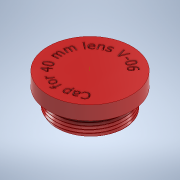
# Autodesk Inventor part: CapForSvBonyPlosse-40mm-V06
Saved by Autodesk Inventor 2021.1 (Build 251245010, 245A)
## iProperties
Created: 2020-10-08
Part Number: CapForSvBonyPlosse-40mm-V06
Material: PC/ABS Plastic
Document SubType Name: Modeling
Designer: robst
Density: 0.357273 g/cm^3
Appearance: Red
Author: robst
Autodesk Inventor part; units mm, degrees
ref_plane "YZ Plane" through (0, 0, 0) normal (1, 0, 0) x (0, 1, 0)
ref_plane "XZ Plane" through (0, 0, 0) normal (0, 1, 0) x (-1, 0, 0)
ref_plane "XY Plane" through (0, 0, 0) normal (0, 0, 1) x (1, 0, 0)
sketch "Sketch7" plane through (0, 0, 0) normal (0, 0, 1) x (1, 0, 0)
  line L0 (0, 0) -> (23.5712, 0)
  line L1 (23.5712, 0) -> (23.5712, 12.7)
  line L2 (23.5712, 12.7) -> (28.575, 12.7)
  line L3 (28.575, 12.7) -> (28.575, 22.225)
  line L4 (28.575, 22.225) -> (0, 22.225)
  line L5 (23.5712, 0) -> (20.3962, 0)
  line L6 (20.3962, 0) -> (20.3962, 19.05)
  line L7 (20.3962, 19.05) -> (12.7, 19.05)
  line L8 (0, 22.225) -> (0, 19.05)
  line L9 (0, -4.445) -> (0, 26.67) projected
  line L10 (0, 19.05) -> (0, 0)
  line L11 (0, 0) -> (12.7, 0)
  line L12 (12.7, 19.05) -> (12.7, 0)
  dimension "d71" = 9.525
  dimension "d72" = 12.7
  dimension "d73" = 23.5712
  dimension "d78" = 3.175
  dimension "d117" = 20.3962
  dimension "d118" = 28.575
  dimension "d122" = 12.7
  constraints: 24 end point, 6 perpendicular, 2 point on line, 2 vertical, 1 collinear, 1 horizontal
  measures "d71" distance between parallel lines of L4 L2
  measures "d72" distance from line of L2 L0.start
  measures "d73" distance of L0.start L0.end
  measures "d78" distance between parallel lines of L1 L6
  measures "d117" distance between parallel lines of L6 L9
  measures "d118" distance from line of L3 L0.start
  measures "d122" distance between parallel lines of L12 L9
revolve "Revolution3" add sketch "Sketch7" angle 360 about axis through (0, -10, 0) along (0, 1, 0) contours L9 L8 L4 L3 L2 L1 L0 L6 L7 L12
sketch "Sketch10" plane through (0, 0, 0) normal (0, 0, 1) x (1, 0, 0)
  line L0 (23.5712, 12.7) -> (23.5712, 0) projected
  line L1 (23.5712, -2.1167) -> (23.5712, -4.0025)
  line L2 (23.5712, -4.0025) -> (22.3266, -3.284)
  line L3 (22.3266, -2.8352) -> (23.5712, -2.1167)
  line L4 (-23.5712, 0) -> (23.5712, 0) projected
  arc A0 (22.3266, -2.8352) -> (22.3266, -3.284) centre (22.4561, -3.0596) ccw
  line L5 (0, -7.3431) -> (0, 16.0405) projected
  point P0 (0, 0)
  dimension "d100" = 60
  dimension "d101" = 2.1167
  dimension "d102" = 0.2591
  dimension "d103" = 22.1971
  constraints: 6 end point, 2 point on circle, 2 tangent, 1 centre point, 1 collinear, 1 equal length, 1 vertical
  measures "d100" angle of L3 L2
  measures "d101" distance from line of L1.start L4
  measures "d102" radius of A0
  measures "d103" distance edge to line of A0 L5
coil "Coil6" sketch "Sketch10" operation cut axis through (0, -10, 0) along (0, 1, 0) pitch 2.1167 turns 8 hand right
sketch "Sketch11" plane through (0, 22.225, 0) normal (0, 1, 0) x (1, 0, 0)
  circle A0 centre (0, 0) radius 20.955 construction
  circle A1 centre (0, 0) radius 28.575 projected
  spline S0 degree 2 poles (11.1336, -14.1453) (11.5615, -13.7907) (12.5248, -13.4798) (13.028, -13.55) knots 0 0 0 1 2 2 2
  spline S1 degree 2 poles (13.028, -13.55) (13.5283, -13.6166) (14.5263, -14.2332) (14.9873, -14.7895) knots 0 0 0 1 2 2 2
  spline S2 degree 2 poles (14.9873, -14.7895) (15.4453, -15.3423) (15.8431, -16.396) (15.8268, -16.9207) knots 0 0 0 1 2 2 2
  spline S3 degree 2 poles (15.8268, -16.9207) (15.8082, -17.4354) (15.3448, -18.3425) (14.8991, -18.7118) knots 0 0 0 1 2 2 2
  spline S4 degree 2 poles (14.8991, -18.7118) (14.678, -18.895) (14.2361, -19.1529) (14.0306, -19.2389) knots 0 0 0 1 2 2 2
  spline S5 degree 2 poles (14.0306, -19.2389) (13.8496, -19.3107) (13.4443, -19.424) (13.233, -19.4667) knots 0 0 0 1 2 2 2
  line L0 (13.233, -19.4667) -> (12.648, -18.7606)
  line L1 (12.648, -18.7606) -> (12.6943, -18.7222)
  spline S6 degree 2 poles (12.6943, -18.7222) (12.8319, -18.7285) (13.2399, -18.7273) (13.4944, -18.6788) knots 0 0 0 1 2 2 2
  spline S7 degree 2 poles (13.4944, -18.6788) (13.7388, -18.6326) (14.2322, -18.4223) (14.489, -18.2096) knots 0 0 0 1 2 2 2
  spline S8 degree 2 poles (14.489, -18.2096) (14.7707, -17.9762) (15.0815, -17.3277) (15.0873, -16.95) knots 0 0 0 1 2 2 2
  spline S9 degree 2 poles (15.0873, -16.95) (15.0866, -16.5717) (14.7291, -15.7192) (14.3774, -15.2948) knots 0 0 0 1 2 2 2
  spline S10 degree 2 poles (14.3774, -15.2948) (14.0022, -14.8419) (13.2439, -14.3695) (12.8688, -14.3014) knots 0 0 0 1 2 2 2
  spline S11 degree 2 poles (12.8688, -14.3014) (12.5031, -14.2375) (11.8242, -14.4272) (11.546, -14.6576) knots 0 0 0 1 2 2 2
  spline S12 degree 2 poles (11.546, -14.6576) (11.2928, -14.8674) (10.9647, -15.3498) (10.8739, -15.5814) knots 0 0 0 1 2 2 2
  spline S13 degree 2 poles (10.8739, -15.5814) (10.7903, -15.807) (10.7109, -16.1976) (10.6993, -16.3215) knots 0 0 0 1 2 2 2
  line L2 (10.6993, -16.3215) -> (10.6565, -16.3569)
  line L3 (10.6565, -16.3569) -> (10.0773, -15.658)
  spline S14 degree 2 poles (10.0773, -15.658) (10.1674, -15.4691) (10.3208, -15.1315) (10.4554, -14.9237) knots 0 0 0 1 2 2 2
  spline S15 degree 2 poles (10.4554, -14.9237) (10.5948, -14.7) (10.8697, -14.364) (11.1336, -14.1453) knots 0 0 0 1 2 2 2
  spline S16 degree 2 poles (7.2823, -17.0834) (7.3335, -16.9868) (7.5001, -16.6496) (7.5951, -16.5267) knots 0 0 0 1 2 2 2
  spline S17 degree 2 poles (7.5951, -16.5267) (7.722, -16.3526) (7.9971, -16.1019) (8.2892, -15.9612) knots 0 0 0 1 2 2 2
  spline S18 degree 2 poles (8.2892, -15.9612) (8.5271, -15.8467) (9.0432, -15.8192) (9.2843, -15.9036) knots 0 0 0 1 2 2 2
  spline S19 degree 2 poles (9.2843, -15.9036) (9.5151, -15.9878) (9.9279, -16.3647) (10.0524, -16.6234) knots 0 0 0 1 2 2 2
  spline S20 degree 2 poles (10.0524, -16.6234) (10.2453, -17.024) (10.1806, -17.7543) (9.8917, -18.0938) knots 0 0 0 1 2 2 2
  spline S21 degree 2 poles (9.8917, -18.0938) (9.6386, -18.4008) (8.8082, -18.9394) (8.309, -19.2157) knots 0 0 0 1 2 2 2
  line L4 (8.309, -19.2157) -> (8.3693, -19.3409)
  spline S22 degree 2 poles (8.3693, -19.3409) (8.4778, -19.5662) (8.7501, -19.7795) (8.9135, -19.7985) knots 0 0 0 1 2 2 2
  spline S23 degree 2 poles (8.9135, -19.7985) (9.0768, -19.8175) (9.4598, -19.6948) (9.6517, -19.6024) knots 0 0 0 1 2 2 2
  spline S24 degree 2 poles (9.6517, -19.6024) (9.8771, -19.4939) (10.422, -19.067) (10.6643, -18.791) knots 0 0 0 1 2 2 2
  line L5 (10.6643, -18.791) -> (10.7019, -18.7729)
  line L6 (10.7019, -18.7729) -> (11.0213, -19.4364)
  spline S25 degree 2 poles (11.0213, -19.4364) (10.866, -19.5728) (10.2545, -20.0215) (9.9248, -20.1802) knots 0 0 0 1 2 2 2
  spline S26 degree 2 poles (9.9248, -20.1802) (9.5242, -20.3731) (8.9173, -20.5111) (8.622, -20.4528) knots 0 0 0 1 2 2 2
  spline S27 degree 2 poles (8.622, -20.4528) (8.3328, -20.3968) (7.8811, -19.9923) (7.7063, -19.6293) knots 0 0 0 1 2 2 2
  line L7 (7.7063, -19.6293) -> (6.4345, -16.9879)
  line L8 (6.4345, -16.9879) -> (7.0854, -16.6745)
  line L9 (7.0854, -16.6745) -> (7.2823, -17.0834)
  line L10 (7.5435, -17.6259) -> (8.0599, -18.6983)
  spline S28 degree 2 poles (8.0599, -18.6983) (8.2835, -18.5649) (8.9546, -18.1544) (9.1436, -17.9812) knots 0 0 0 1 2 2 2
  spline S29 degree 2 poles (9.1436, -17.9812) (9.3641, -17.7773) (9.5434, -17.2849) (9.4027, -16.9928) knots 0 0 0 1 2 2 2
  spline S30 degree 2 poles (9.4027, -16.9928) (9.242, -16.659) (8.7037, -16.5018) (8.3448, -16.6746) knots 0 0 0 1 2 2 2
  spline S31 degree 2 poles (8.3448, -16.6746) (8.0402, -16.8213) (7.6661, -17.3253) (7.5435, -17.6259) knots 0 0 0 1 2 2 2
  spline S32 degree 2 poles (2.4585, -20.302) (2.2284, -19.2524) (2.9565, -17.7937) (3.7211, -17.6262) knots 0 0 0 1 2 2 2
  spline S33 degree 2 poles (3.7211, -17.6262) (4.0332, -17.5578) (4.5445, -17.5974) (4.826, -17.6922) knots 0 0 0 1 2 2 2
  line L11 (4.826, -17.6922) -> (4.4413, -15.9369)
  line L12 (4.4413, -15.9369) -> (5.147, -15.7822)
  line L13 (5.147, -15.7822) -> (6.4033, -21.514)
  line L14 (6.4033, -21.514) -> (5.6976, -21.6687)
  line L15 (5.6976, -21.6687) -> (5.6014, -21.2299)
  spline S34 degree 2 poles (5.6014, -21.2299) (5.3916, -21.5271) (4.8186, -21.9846) (4.4431, -22.0669) knots 0 0 0 1 2 2 2
  spline S35 degree 2 poles (4.4431, -22.0669) (3.7238, -22.2246) (2.6687, -21.261) (2.4585, -20.302) knots 0 0 0 1 2 2 2
  spline S36 degree 2 poles (3.169, -20.0609) (3.3266, -20.7802) (3.9571, -21.4717) (4.4683, -21.3597) knots 0 0 0 1 2 2 2
  spline S37 degree 2 poles (4.4683, -21.3597) (4.7668, -21.2942) (5.2693, -20.9044) (5.4725, -20.6418) knots 0 0 0 1 2 2 2
  line L16 (5.4725, -20.6418) -> (4.9509, -18.2622)
  spline S38 degree 2 poles (4.9509, -18.2622) (4.6462, -18.1915) (4.2308, -18.1782) (3.9775, -18.2337) knots 0 0 0 1 2 2 2
  spline S39 degree 2 poles (3.9775, -18.2337) (3.4301, -18.3537) (3.0004, -19.2918) (3.169, -20.0609) knots 0 0 0 1 2 2 2
  line L17 (-4.0637, -23.0619) -> (-4.0269, -23.066)
  spline S40 degree 2 poles (-4.0269, -23.066) (-3.9344, -23.1138) (-3.5827, -23.2188) (-3.4401, -23.235) knots 0 0 0 1 2 2 2
  spline S41 degree 2 poles (-3.4401, -23.235) (-2.9891, -23.286) (-2.5567, -22.9248) (-2.4963, -22.3909) knots 0 0 0 1 2 2 2
  line L18 (-2.4963, -22.3909) -> (-2.4802, -22.2483)
  line L19 (-2.4802, -22.2483) -> (-3.6675, -22.1139)
  line L20 (-3.6675, -22.1139) -> (-3.6003, -21.5203)
  line L21 (-3.6003, -21.5203) -> (-2.436, -21.652)
  line L22 (-2.436, -21.652) -> (-2.021, -17.9843)
  line L23 (-2.021, -17.9843) -> (-1.3031, -18.0655)
  line L24 (-1.3031, -18.0655) -> (-1.7181, -21.7333)
  line L25 (-1.7181, -21.7333) -> (-1.2349, -21.7879)
  line L26 (-1.2349, -21.7879) -> (-1.3021, -22.3816)
  line L27 (-1.3021, -22.3816) -> (-1.7853, -22.3269)
  line L28 (-1.7853, -22.3269) -> (-1.8014, -22.4696)
  spline S42 degree 2 poles (-1.8014, -22.4696) (-1.8878, -23.2335) (-2.7194, -23.9504) (-3.4096, -23.8723) knots 0 0 0 1 2 2 2
  spline S43 degree 2 poles (-3.4096, -23.8723) (-3.6075, -23.8499) (-3.9848, -23.7653) (-4.1381, -23.7199) knots 0 0 0 1 2 2 2
  line L29 (-4.1381, -23.7199) -> (-4.0637, -23.0619)
  spline S44 degree 2 poles (-7.8779, -18.744) (-7.5539, -17.7098) (-6.2065, -16.8943) (-5.3757, -17.1545) knots 0 0 0 1 2 2 2
  spline S45 degree 2 poles (-5.3757, -17.1545) (-4.5227, -17.4217) (-3.91, -18.89) (-4.2229, -19.8888) knots 0 0 0 1 2 2 2
  spline S46 degree 2 poles (-4.2229, -19.8888) (-4.5441, -20.9141) (-5.9075, -21.7343) (-6.7295, -21.4769) knots 0 0 0 1 2 2 2
  spline S47 degree 2 poles (-6.7295, -21.4769) (-7.5604, -21.2166) (-8.2004, -19.7737) (-7.8779, -18.744) knots 0 0 0 1 2 2 2
  spline S48 degree 2 poles (-7.1663, -18.9668) (-7.4155, -19.7624) (-7.0788, -20.7171) (-6.544, -20.8846) knots 0 0 0 1 2 2 2
  spline S49 degree 2 poles (-6.544, -20.8846) (-6.0093, -21.0521) (-5.1836, -20.4614) (-4.9344, -19.6659) knots 0 0 0 1 2 2 2
  spline S50 degree 2 poles (-4.9344, -19.6659) (-4.6922, -18.8925) (-5.0264, -17.9143) (-5.5612, -17.7468) knots 0 0 0 1 2 2 2
  spline S51 degree 2 poles (-5.5612, -17.7468) (-6.0915, -17.5806) (-6.9199, -18.1802) (-7.1663, -18.9668) knots 0 0 0 1 2 2 2
  line L30 (-11.5545, -18.3168) -> (-11.5219, -18.3345)
  spline S52 degree 2 poles (-11.5219, -18.3345) (-11.4598, -18.3948) (-11.3057, -18.4893) (-11.1959, -18.5492) knots 0 0 0 1 2 2 2
  spline S53 degree 2 poles (-11.1959, -18.5492) (-10.9397, -18.6888) (-10.3135, -18.7399) (-9.9661, -18.6445) knots 0 0 0 1 2 2 2
  line L31 (-9.9661, -18.6445) -> (-8.51, -15.9727)
  line L32 (-8.51, -15.9727) -> (-7.8756, -16.3185)
  line L33 (-7.8756, -16.3185) -> (-9.9279, -20.0841)
  line L34 (-9.9279, -20.0841) -> (-10.5623, -19.7384)
  line L35 (-10.5623, -19.7384) -> (-10.2564, -19.1772)
  spline S54 degree 2 poles (-10.2564, -19.1772) (-10.7705, -19.2979) (-11.4244, -19.2685) (-11.6684, -19.1355) knots 0 0 0 1 2 2 2
  spline S55 degree 2 poles (-11.6684, -19.1355) (-11.766, -19.0823) (-11.8592, -19.021) (-11.9135, -18.9756) knots 0 0 0 1 2 2 2
  line L36 (-11.9135, -18.9756) -> (-11.5545, -18.3168)
  line L37 (-16.1257, -12.0919) -> (-15.6665, -12.5945)
  line L38 (-15.6665, -12.5945) -> (-14.2168, -11.27)
  line L39 (-14.2168, -11.27) -> (-13.7201, -11.8136)
  line L40 (-13.7201, -11.8136) -> (-15.1698, -13.1381)
  line L41 (-15.1698, -13.1381) -> (-13.4674, -15.0016)
  line L42 (-13.4674, -15.0016) -> (-14.0623, -15.5451)
  line L43 (-14.0623, -15.5451) -> (-17.9612, -15.6445)
  line L44 (-17.9612, -15.6445) -> (-18.436, -15.1248)
  line L45 (-18.436, -15.1248) -> (-16.1213, -13.0099)
  line L46 (-16.1213, -13.0099) -> (-16.5805, -12.5073)
  line L47 (-16.5805, -12.5073) -> (-16.1257, -12.0919)
  line L48 (-15.6246, -13.5536) -> (-17.2726, -15.0593)
  line L49 (-17.2726, -15.0593) -> (-14.3282, -14.9725)
  line L50 (-14.3282, -14.9725) -> (-15.6246, -13.5536)
  spline S56 degree 2 poles (-19.2293, -8.5261) (-17.8832, -7.7829) (-16.1903, -7.8693) (-15.7404, -8.6843) knots 0 0 0 1 2 2 2
  spline S57 degree 2 poles (-15.7404, -8.6843) (-15.2837, -9.5114) (-16.1415, -10.9953) (-17.4592, -11.7228) knots 0 0 0 1 2 2 2
  spline S58 degree 2 poles (-17.4592, -11.7228) (-18.8134, -12.4704) (-20.4982, -12.3795) (-20.9504, -11.5605) knots 0 0 0 1 2 2 2
  spline S59 degree 2 poles (-20.9504, -11.5605) (-21.4047, -10.7374) (-20.5348, -9.2468) (-19.2293, -8.5261) knots 0 0 0 1 2 2 2
  spline S60 degree 2 poles (-17.2303, -8.544) (-17.5313, -8.5832) (-18.3383, -8.9229) (-18.8532, -9.2072) knots 0 0 0 1 2 2 2
  spline S61 degree 2 poles (-18.8532, -9.2072) (-19.3682, -9.4915) (-20.0816, -9.9911) (-20.2811, -10.2335) knots 0 0 0 1 2 2 2
  spline S62 degree 2 poles (-20.2811, -10.2335) (-20.4805, -10.4759) (-20.5493, -10.9741) (-20.3949, -11.2539) knots 0 0 0 1 2 2 2
  spline S63 degree 2 poles (-20.3949, -11.2539) (-20.2405, -11.5336) (-19.7777, -11.749) (-19.456, -11.7089) knots 0 0 0 1 2 2 2
  spline S64 degree 2 poles (-19.456, -11.7089) (-19.1446, -11.6693) (-18.3258, -11.3125) (-17.8352, -11.0416) knots 0 0 0 1 2 2 2
  spline S65 degree 2 poles (-17.8352, -11.0416) (-17.3082, -10.7507) (-16.6385, -10.2963) (-16.421, -10.0387) knots 0 0 0 1 2 2 2
  spline S66 degree 2 poles (-16.421, -10.0387) (-16.2152, -9.7981) (-16.1347, -9.2829) (-16.2958, -8.9909) knots 0 0 0 1 2 2 2
  spline S67 degree 2 poles (-16.2958, -8.9909) (-16.448, -8.7152) (-16.9108, -8.4999) (-17.2303, -8.544) knots 0 0 0 1 2 2 2
  line L51 (-18.1997, 0.8026) -> (-20.6758, 0.6272)
  spline S68 degree 2 poles (-20.6758, 0.6272) (-20.9715, 0.6062) (-21.4718, 0.5244) (-21.6051, 0.4407) knots 0 0 0 1 2 2 2
  spline S69 degree 2 poles (-21.6051, 0.4407) (-21.7524, 0.3559) (-21.8802, 0.0637) (-21.8629, -0.1812) knots 0 0 0 1 2 2 2
  spline S70 degree 2 poles (-21.8629, -0.1812) (-21.8472, -0.4029) (-21.5386, -0.8918) (-21.2609, -1.1414) knots 0 0 0 1 2 2 2
  spline S71 degree 2 poles (-21.2609, -1.1414) (-21.1966, -1.1322) (-21.0171, -1.1102) (-20.897, -1.1017) knots 0 0 0 1 2 2 2
  line L52 (-20.897, -1.1017) -> (-18.0789, -0.9021)
  line L53 (-18.0789, -0.9021) -> (-18.0279, -1.6228)
  line L54 (-18.0279, -1.6228) -> (-20.5041, -1.7982)
  spline S72 degree 2 poles (-20.5041, -1.7982) (-20.7997, -1.8191) (-21.3, -1.901) (-21.4334, -1.9847) knots 0 0 0 1 2 2 2
  spline S73 degree 2 poles (-21.4334, -1.9847) (-21.5806, -2.0694) (-21.7084, -2.3617) (-21.6911, -2.6065) knots 0 0 0 1 2 2 2
  spline S74 degree 2 poles (-21.6911, -2.6065) (-21.6747, -2.8375) (-21.3474, -3.3297) (-21.104, -3.5539) knots 0 0 0 1 2 2 2
  line L55 (-21.104, -3.5539) -> (-17.9072, -3.3274)
  line L56 (-17.9072, -3.3274) -> (-17.8561, -4.0481)
  line L57 (-17.8561, -4.0481) -> (-22.134, -4.3511)
  line L58 (-22.134, -4.3511) -> (-22.185, -3.6304)
  line L59 (-22.185, -3.6304) -> (-21.7138, -3.5971)
  spline S75 degree 2 poles (-21.7138, -3.5971) (-22.0156, -3.3352) (-22.3643, -2.8028) (-22.3879, -2.4702) knots 0 0 0 1 2 2 2
  spline S76 degree 2 poles (-22.3879, -2.4702) (-22.4147, -2.0913) (-22.1098, -1.4801) (-21.7279, -1.2998) knots 0 0 0 1 2 2 2
  spline S77 degree 2 poles (-21.7279, -1.2998) (-22.1161, -0.9977) (-22.5342, -0.4052) (-22.5597, -0.0448) knots 0 0 0 1 2 2 2
  spline S78 degree 2 poles (-22.5597, -0.0448) (-22.5793, 0.2324) (-22.4405, 0.6972) (-22.2582, 0.8773) knots 0 0 0 1 2 2 2
  spline S79 degree 2 poles (-22.2582, 0.8773) (-22.0763, 1.0619) (-21.5076, 1.2926) (-21.0687, 1.3236) knots 0 0 0 1 2 2 2
  line L60 (-21.0687, 1.3236) -> (-18.2507, 1.5232)
  line L61 (-18.2507, 1.5232) -> (-18.1997, 0.8026)
  line L62 (-16.7452, 7.1742) -> (-19.124, 7.884)
  spline S80 degree 2 poles (-19.124, 7.884) (-19.408, 7.9688) (-19.905, 8.0688) (-20.0593, 8.0375) knots 0 0 0 1 2 2 2
  spline S81 degree 2 poles (-20.0593, 8.0375) (-20.2269, 8.0102) (-20.4497, 7.7819) (-20.5199, 7.5466) knots 0 0 0 1 2 2 2
  spline S82 degree 2 poles (-20.5199, 7.5466) (-20.5835, 7.3336) (-20.4673, 6.7673) (-20.2956, 6.4358) knots 0 0 0 1 2 2 2
  spline S83 degree 2 poles (-20.2956, 6.4358) (-20.2321, 6.4217) (-20.0564, 6.3789) (-19.941, 6.3445) knots 0 0 0 1 2 2 2
  line L63 (-19.941, 6.3445) -> (-17.2339, 5.5366)
  line L64 (-17.2339, 5.5366) -> (-17.4405, 4.8443)
  line L65 (-17.4405, 4.8443) -> (-19.8192, 5.5541)
  spline S84 degree 2 poles (-19.8192, 5.5541) (-20.1032, 5.6389) (-20.6002, 5.7389) (-20.7545, 5.7076) knots 0 0 0 1 2 2 2
  spline S85 degree 2 poles (-20.7545, 5.7076) (-20.9222, 5.6803) (-21.145, 5.452) (-21.2152, 5.2167) knots 0 0 0 1 2 2 2
  spline S86 degree 2 poles (-21.2152, 5.2167) (-21.2814, 4.9948) (-21.1488, 4.4188) (-21.0002, 4.1231) knots 0 0 0 1 2 2 2
  line L66 (-21.0002, 4.1231) -> (-17.9292, 3.2067)
  line L67 (-17.9292, 3.2067) -> (-18.1358, 2.5144)
  line L68 (-18.1358, 2.5144) -> (-22.2453, 3.7407)
  line L69 (-22.2453, 3.7407) -> (-22.0387, 4.433)
  line L70 (-22.0387, 4.433) -> (-21.586, 4.298)
  spline S87 degree 2 poles (-21.586, 4.298) (-21.7759, 4.6495) (-21.9144, 5.2707) (-21.819, 5.5903) knots 0 0 0 1 2 2 2
  spline S88 degree 2 poles (-21.819, 5.5903) (-21.7104, 5.9542) (-21.2094, 6.4185) (-20.7885, 6.4523) knots 0 0 0 1 2 2 2
  spline S89 degree 2 poles (-20.7885, 6.4523) (-21.045, 6.8721) (-21.227, 7.574) (-21.1237, 7.9202) knots 0 0 0 1 2 2 2
  spline S90 degree 2 poles (-21.1237, 7.9202) (-21.0443, 8.1864) (-20.7503, 8.5723) (-20.5162, 8.6765) knots 0 0 0 1 2 2 2
  spline S91 degree 2 poles (-20.5162, 8.6765) (-20.2808, 8.7851) (-19.6674, 8.8002) (-19.2458, 8.6744) knots 0 0 0 1 2 2 2
  line L71 (-19.2458, 8.6744) -> (-16.5387, 7.8665)
  line L72 (-16.5387, 7.8665) -> (-16.7452, 7.1742)
  line L73 (-14.1279, 11.3161) -> (-14.5682, 10.7433)
  line L74 (-14.5682, 10.7433) -> (-19.3011, 14.3816)
  line L75 (-19.3011, 14.3816) -> (-18.8608, 14.9544)
  line L76 (-18.8608, 14.9544) -> (-14.1279, 11.3161)
  spline S92 degree 2 poles (-12.0649, 13.3622) (-12.8157, 12.6598) (-14.4288, 12.73) (-15.1564, 13.5079) knots 0 0 0 1 2 2 2
  spline S93 degree 2 poles (-15.1564, 13.5079) (-15.8715, 14.2723) (-15.9178, 15.9285) (-15.2718, 16.5328) knots 0 0 0 1 2 2 2
  spline S94 degree 2 poles (-15.2718, 16.5328) (-14.9809, 16.8049) (-14.3729, 17.0566) (-14.0395, 17.0324) knots 0 0 0 1 2 2 2
  spline S95 degree 2 poles (-14.0395, 17.0324) (-13.7027, 17.0113) (-13.0394, 16.6615) (-12.6882, 16.2861) knots 0 0 0 1 2 2 2
  line L77 (-12.6882, 16.2861) -> (-12.4193, 15.9986)
  line L78 (-12.4193, 15.9986) -> (-14.5873, 13.9706)
  spline S96 degree 2 poles (-14.5873, 13.9706) (-14.0779, 13.4261) (-12.989, 13.3602) (-12.5019, 13.8158) knots 0 0 0 1 2 2 2
  spline S97 degree 2 poles (-12.5019, 13.8158) (-12.3294, 13.9772) (-12.0674, 14.3682) (-11.989, 14.5556) knots 0 0 0 1 2 2 2
  spline S98 degree 2 poles (-11.989, 14.5556) (-11.9103, 14.7561) (-11.8248, 15.058) (-11.8112, 15.1722) knots 0 0 0 1 2 2 2
  line L79 (-11.8112, 15.1722) -> (-11.7807, 15.2007)
  line L80 (-11.7807, 15.2007) -> (-11.2429, 14.6257)
  spline S99 degree 2 poles (-11.2429, 14.6257) (-11.2994, 14.5031) (-11.4755, 14.1355) (-11.5553, 14.0038) knots 0 0 0 1 2 2 2
  spline S100 degree 2 poles (-11.5553, 14.0038) (-11.6663, 13.8174) (-11.8755, 13.5393) (-12.0649, 13.3622) knots 0 0 0 1 2 2 2
  spline S101 degree 2 poles (-13.3099, 15.9202) (-13.5159, 16.1269) (-13.8949, 16.3558) (-14.0776, 16.3816) knots 0 0 0 1 2 2 2
  spline S102 degree 2 poles (-14.0776, 16.3816) (-14.2796, 16.4145) (-14.6842, 16.2707) (-14.8973, 16.0714) knots 0 0 0 1 2 2 2
  spline S103 degree 2 poles (-14.8973, 16.0714) (-15.107, 15.8753) (-15.2841, 15.4749) (-15.292, 15.2392) knots 0 0 0 1 2 2 2
  spline S104 degree 2 poles (-15.292, 15.2392) (-15.2933, 15.0034) (-15.1335, 14.5884) (-14.9638, 14.3731) knots 0 0 0 1 2 2 2
  line L81 (-14.9638, 14.3731) -> (-13.3099, 15.9202)
  line L82 (-7.4811, 16.5663) -> (-8.1089, 16.2086)
  line L83 (-8.1089, 16.2086) -> (-9.3193, 18.3334)
  spline S105 degree 2 poles (-9.3193, 18.3334) (-9.466, 18.5909) (-9.7665, 19.0061) (-9.9146, 19.0976) knots 0 0 0 1 2 2 2
  spline S106 degree 2 poles (-9.9146, 19.0976) (-10.0712, 19.1949) (-10.4228, 19.1758) (-10.6562, 19.0429) knots 0 0 0 1 2 2 2
  spline S107 degree 2 poles (-10.6562, 19.0429) (-10.8896, 18.9099) (-11.2425, 18.3784) (-11.3653, 18.042) knots 0 0 0 1 2 2 2
  line L84 (-11.3653, 18.042) -> (-9.7789, 15.2573)
  line L85 (-9.7789, 15.2573) -> (-10.4067, 14.8997)
  line L86 (-10.4067, 14.8997) -> (-12.5295, 18.626)
  line L87 (-12.5295, 18.626) -> (-11.9017, 18.9836)
  line L88 (-11.9017, 18.9836) -> (-11.6656, 18.5691)
  spline S108 degree 2 poles (-11.6656, 18.5691) (-11.5283, 18.9831) (-11.1364, 19.5582) (-10.8305, 19.7324) knots 0 0 0 1 2 2 2
  spline S109 degree 2 poles (-10.8305, 19.7324) (-10.2832, 20.0442) (-9.2509, 19.6729) (-8.8589, 18.9848) knots 0 0 0 1 2 2 2
  line L89 (-8.8589, 18.9848) -> (-7.4811, 16.5663)
  spline S110 degree 2 poles (-5.4004, 17.1663) (-5.8118, 17.0387) (-6.5925, 17.039) (-6.8654, 17.0901) knots 0 0 0 1 2 2 2
  line L90 (-6.8654, 17.0901) -> (-7.1055, 17.8642)
  line L91 (-7.1055, 17.8642) -> (-7.0701, 17.8752)
  spline S111 degree 2 poles (-7.0701, 17.8752) (-6.9597, 17.8318) (-6.6687, 17.7378) (-6.4408, 17.7067) knots 0 0 0 1 2 2 2
  spline S112 degree 2 poles (-6.4408, 17.7067) (-6.2423, 17.6762) (-5.7792, 17.684) (-5.5536, 17.754) knots 0 0 0 1 2 2 2
  spline S113 degree 2 poles (-5.5536, 17.754) (-5.3899, 17.8048) (-5.0373, 17.9966) (-4.968, 18.086) knots 0 0 0 1 2 2 2
  spline S114 degree 2 poles (-4.968, 18.086) (-4.8658, 18.2098) (-4.8098, 18.4357) (-4.8702, 18.6303) knots 0 0 0 1 2 2 2
  spline S115 degree 2 poles (-4.8702, 18.6303) (-4.9457, 18.8736) (-5.2893, 19.0434) (-5.6559, 19.0218) knots 0 0 0 1 2 2 2
  spline S116 degree 2 poles (-5.6559, 19.0218) (-5.7982, 19.0116) (-6.2503, 18.9683) (-6.4468, 18.9607) knots 0 0 0 1 2 2 2
  spline S117 degree 2 poles (-6.4468, 18.9607) (-6.9582, 18.9524) (-7.5585, 19.3869) (-7.6833, 19.7894) knots 0 0 0 1 2 2 2
  spline S118 degree 2 poles (-7.6833, 19.7894) (-7.8562, 20.3467) (-7.2357, 21.3005) (-6.5456, 21.5146) knots 0 0 0 1 2 2 2
  spline S119 degree 2 poles (-6.5456, 21.5146) (-6.205, 21.6203) (-5.4628, 21.6662) (-5.1886, 21.6107) knots 0 0 0 1 2 2 2
  line L92 (-5.1886, 21.6107) -> (-4.9595, 20.872)
  line L93 (-4.9595, 20.872) -> (-4.9948, 20.861)
  spline S120 degree 2 poles (-4.9948, 20.861) (-5.3261, 20.991) (-6.0474, 21.0339) (-6.3791, 20.931) knots 0 0 0 1 2 2 2
  spline S121 degree 2 poles (-6.3791, 20.931) (-6.7197, 20.8254) (-7.0994, 20.3924) (-7.0102, 20.1049) knots 0 0 0 1 2 2 2
  spline S122 degree 2 poles (-7.0102, 20.1049) (-6.9293, 19.8439) (-6.5724, 19.6782) (-6.238, 19.6947) knots 0 0 0 1 2 2 2
  spline S123 degree 2 poles (-6.238, 19.6947) (-6.0753, 19.7015) (-5.6702, 19.7399) (-5.4472, 19.7557) knots 0 0 0 1 2 2 2
  spline S124 degree 2 poles (-5.4472, 19.7557) (-4.9603, 19.7807) (-4.337, 19.397) (-4.1957, 18.9414) knots 0 0 0 1 2 2 2
  spline S125 degree 2 poles (-4.1957, 18.9414) (-4.1134, 18.676) (-4.1758, 18.1426) (-4.3258, 17.907) knots 0 0 0 1 2 2 2
  spline S126 degree 2 poles (-4.3258, 17.907) (-4.4863, 17.6584) (-4.9802, 17.2967) (-5.4004, 17.1663) knots 0 0 0 1 2 2 2
  line L94 (3.8129, 23.622) -> (1.4952, 18.0396)
  line L95 (1.4952, 18.0396) -> (0.677, 18.0902)
  line L96 (0.677, 18.0902) -> (-0.9343, 23.916)
  line L97 (-0.9343, 23.916) -> (-0.1207, 23.8656)
  line L98 (-0.1207, 23.8656) -> (1.1667, 19.0297)
  line L99 (1.1667, 19.0297) -> (3.041, 23.6698)
  line L100 (3.041, 23.6698) -> (3.8129, 23.622)
  line L101 (6.4683, 19.2208) -> (4.3845, 19.8001)
  line L102 (4.3845, 19.8001) -> (4.5706, 20.4694)
  line L103 (4.5706, 20.4694) -> (6.6544, 19.8901)
  line L104 (6.6544, 19.8901) -> (6.4683, 19.2208)
  spline S127 degree 2 poles (11.081, 17.8793) (10.3878, 16.5069) (8.9405, 15.6243) (8.1096, 16.044) knots 0 0 0 1 2 2 2
  spline S128 degree 2 poles (8.1096, 16.044) (7.2663, 16.47) (7.1387, 18.1792) (7.8174, 19.5227) knots 0 0 0 1 2 2 2
  spline S129 degree 2 poles (7.8174, 19.5227) (8.5148, 20.9034) (9.9579, 21.7777) (10.7929, 21.3559) knots 0 0 0 1 2 2 2
  spline S130 degree 2 poles (10.7929, 21.3559) (11.6321, 20.932) (11.7534, 19.2104) (11.081, 17.8793) knots 0 0 0 1 2 2 2
  spline S131 degree 2 poles (9.4195, 16.7677) (9.6461, 16.9697) (10.1214, 17.7051) (10.3866, 18.2301) knots 0 0 0 1 2 2 2
  spline S132 degree 2 poles (10.3866, 18.2301) (10.6518, 18.7551) (10.9596, 19.5699) (10.9878, 19.8825) knots 0 0 0 1 2 2 2
  spline S133 degree 2 poles (10.9878, 19.8825) (11.016, 20.1951) (10.7921, 20.6455) (10.5068, 20.7896) knots 0 0 0 1 2 2 2
  spline S134 degree 2 poles (10.5068, 20.7896) (10.2216, 20.9337) (9.718, 20.8508) (9.4748, 20.6364) knots 0 0 0 1 2 2 2
  spline S135 degree 2 poles (9.4748, 20.6364) (9.2399, 20.4282) (8.7645, 19.6721) (8.5119, 19.1719) knots 0 0 0 1 2 2 2
  spline S136 degree 2 poles (8.5119, 19.1719) (8.2404, 18.6345) (7.9432, 17.8818) (7.9087, 17.5464) knots 0 0 0 1 2 2 2
  spline S137 degree 2 poles (7.9087, 17.5464) (7.8743, 17.2317) (8.0981, 16.7607) (8.3957, 16.6103) knots 0 0 0 1 2 2 2
  spline S138 degree 2 poles (8.3957, 16.6103) (8.6768, 16.4683) (9.1805, 16.5512) (9.4195, 16.7677) knots 0 0 0 1 2 2 2
  spline S139 degree 2 poles (14.3446, 13.9924) (14.0599, 13.657) (13.355, 13.2772) (13.0061, 13.2453) knots 0 0 0 1 2 2 2
  spline S140 degree 2 poles (13.0061, 13.2453) (12.6411, 13.2088) (11.9769, 13.414) (11.6838, 13.6627) knots 0 0 0 1 2 2 2
  spline S141 degree 2 poles (11.6838, 13.6627) (11.3907, 13.9114) (11.0747, 14.5196) (11.0589, 14.8732) knots 0 0 0 1 2 2 2
  spline S142 degree 2 poles (11.0589, 14.8732) (11.0337, 15.3016) (11.4536, 16.3118) (11.945, 16.891) knots 0 0 0 1 2 2 2
  spline S143 degree 2 poles (11.945, 16.891) (12.4274, 17.4595) (13.4365, 18.1764) (13.9678, 18.3087) knots 0 0 0 1 2 2 2
  spline S144 degree 2 poles (13.9678, 18.3087) (14.4861, 18.4399) (15.5494, 18.1754) (16.0402, 17.7589) knots 0 0 0 1 2 2 2
  spline S145 degree 2 poles (16.0402, 17.7589) (16.185, 17.6361) (16.4153, 17.3921) (16.4837, 17.2794) knots 0 0 0 1 2 2 2
  line L105 (16.4837, 17.2794) -> (16.0073, 16.7179)
  line L106 (16.0073, 16.7179) -> (15.9825, 16.7389)
  spline S146 degree 2 poles (15.9825, 16.7389) (15.9373, 16.8502) (15.7036, 17.176) (15.5341, 17.3199) knots 0 0 0 1 2 2 2
  spline S147 degree 2 poles (15.5341, 17.3199) (14.9902, 17.7813) (13.6996, 17.6131) (13.0247, 16.9466) knots 0 0 0 1 2 2 2
  spline S148 degree 2 poles (13.0247, 16.9466) (13.3559, 16.9146) (13.9287, 16.702) (14.19, 16.4803) knots 0 0 0 1 2 2 2
  spline S149 degree 2 poles (14.19, 16.4803) (14.4442, 16.2645) (14.7387, 15.8385) (14.8152, 15.5063) knots 0 0 0 1 2 2 2
  spline S150 degree 2 poles (14.8152, 15.5063) (14.9026, 15.1225) (14.6622, 14.3668) (14.3446, 13.9924) knots 0 0 0 1 2 2 2
  spline S151 degree 2 poles (13.7303, 14.4711) (13.9581, 14.7395) (14.1254, 15.2231) (14.0779, 15.4821) knots 0 0 0 1 2 2 2
  spline S152 degree 2 poles (14.0779, 15.4821) (14.0393, 15.6728) (13.8007, 15.9785) (13.6488, 16.1073) knots 0 0 0 1 2 2 2
  spline S153 degree 2 poles (13.6488, 16.1073) (13.444, 16.2811) (12.9542, 16.4841) (12.6682, 16.5264) knots 0 0 0 1 2 2 2
  spline S154 degree 2 poles (12.6682, 16.5264) (12.6107, 16.4658) (12.5018, 16.3518) (12.4239, 16.2599) knots 0 0 0 1 2 2 2
  spline S155 degree 2 poles (12.4239, 16.2599) (12.0403, 15.8079) (11.7465, 15.1037) (11.7578, 14.845) knots 0 0 0 1 2 2 2
  spline S156 degree 2 poles (11.7578, 14.845) (11.7645, 14.6024) (11.94, 14.2652) (12.0919, 14.1364) knots 0 0 0 1 2 2 2
  spline S157 degree 2 poles (12.0919, 14.1364) (12.445, 13.8368) (13.3049, 13.9697) (13.7303, 14.4711) knots 0 0 0 1 2 2 2
  dimension "d121" = 7.62
  constraints: 1 centre point, 1 coincident, 1 other
  measures "d121" radial gap between concentric circles of A0 A1
extrude "Extrusion1" cut sketch "Sketch11" against normal blind 1.905 contours S0 S1 S2 S3 S4 S5 L0 L1 S6 S7 S8 S9 S10 S11 S12 S13 L2 L3 S14 S15 | S16 S17 S18 S19 S20 S21 L4 S22 S23 S24 L5 L6 S25 S26 S27 L7 L8 L9 | S32 S33 L11 L12 L13 L14 L15 S34 S35 | L17 S40 S41 L18 L19 L20 L21 L22 L23 L24 L25 L26 L27 L28 S42 S43 L29 | S44 S45 S46 S47 | L30 S52 S53 L31 L32 L33 L34 L35 S54 S55 L36 | L37 L38 L39 L40 L41 L42 L43 L44 L45 L46 L47 | S56 S57 S58 S59 | L51 S68 S69 S70 S71 L52 L53 L54 S72 S73 S74 L55 L56 L57 L58 L59 S75 S76 S77 S78 S79 L60 L61 | L62 S80 S81 S82 S83 L63 L64 L65 S84 S85 S86 L66 L67 L68 L69 L70 S87 S88 S89 S90 S91 L71 L72 | L73 L74 L75 L76 | S92 S93 S94 S95 L77 L78 S96 S97 S98 L79 L80 S99 S100 | L82 L83 S105 S106 S107 L84 L85 L86 L87 L88 S108 S109 L89 | S110 L90 L91 S111 S112 S113 S114 S115 S116 S117 S118 S119 L92 L93 S120 S121 S122 S123 S124 S125 S126 | L94 L95 L96 L97 L98 L99 L100 | L101 L102 L103 L104 | S127 S128 S129 S130 | S139 S140 S141 S142 S143 S144 S145 L105 L106 S146 S147 S148 S149 S150
equation "\"d72\" = caseHeightAboveLens"
equation "\"d73\" = a1MajorRadius"
equation "\"d78\" = wallThickness"
equation "\"d118\" = capExteriorRadius"
equation "\"d122\" = innerPostRadius"
equation "\"d100\" = threadAngle"
equation "\"d101\" = pitch"
equation "\"d102\" = a1RootRadius"
equation "\"d103\" = a1MinorRadius"
equation "\"d104\" = pitch"
equation "\"baseDiameter\" = 31.75"
equation "\"baseRadius\" = 0.5 * baseDiameter"
equation "\"baseHeight\" = 25.4"
equation "\"middleDiameter\" = 34.29"
equation "\"middleRadius\" = 0.5 * middleDiameter"
equation "\"middleTopDiameter\" = 34.798"
equation "\"middleTopRadius\" = 0.5 * middleTopDiameter"
equation "\"middleHeight\" = 18.542"
equation "\"middleTopHeight\" = 30.734"
equation "\"topBaseDiameter\" = 34.798"
equation "\"topHeightDiameter\" = 40.894"
equation "\"topBaseRadius\" = 0.5 * topBaseDiameter"
equation "\"topHeightRadius\" = 0.5 * topHeightDiameter"
equation "\"topHeight\" = 7.62"
equation "\"d9\" = caseBottomThickness"
equation "\"wallThickness\" = 3.175"
equation "\"caseBottomThickness\" = 4.7625"
equation "\"caseHeightAboveLens\" = 12.7"
equation "\"baseWallThickness\" = 2.032"
equation "\"baseInteriorHeight\" = 15.24"
equation "\"interiorDiameter\" = 41.275"
equation "\"interiorRadius\" = 0.5 * interiorDiameter"
equation "\"outsideRadius\" = interiorRadius + wallThickness"
equation "\"outsideDiameter\" = 2 * outsideRadius"
equation "\"textRingDiameter\" = 0.75 * outsideDiameter"
equation "\"b2MajorDiameterMax\" = 41.275"
equation "\"b2MajorRadiusMax\" = 0.5 * b2MajorDiameterMax"
equation "\"a1MinorDiameter\" = 44.39412"
equation "\"a1MinorRadius\" = 0.5 * a1MinorDiameter"
equation "\"a1MajorDiameter\" = 47.1424"
equation "\"a1MajorRadius\" = 0.5 * a1MajorDiameter"
equation "\"a1RootRadius\" = 0.25908"
equation "\"topThickness\" = 9.525"
equation "\"threadAngle\" = 60deg"
equation "\"capExteriorDiameter\" = 57.15"
equation "\"capExteriorRadius\" = 0.5 * capExteriorDiameter"
equation "\"innerPostDiameter\" = 25.4"
equation "\"innerPostRadius\" = 0.5 * innerPostDiameter"
equation "\"pitch\" = 2.116667"
body "Solid3"
